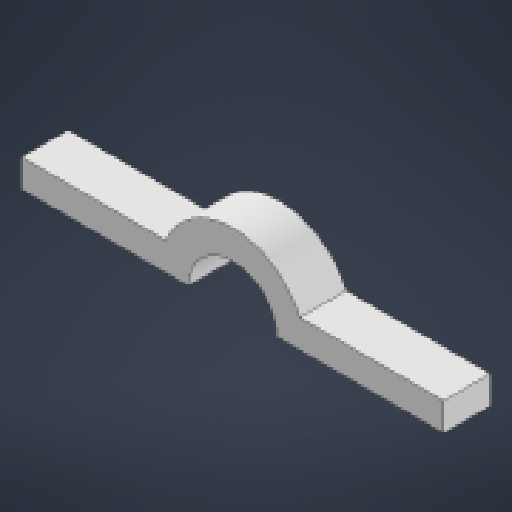
# Autodesk Inventor part: Idler-Clamp
Saved by Autodesk Inventor 2025 (Build 290162010, 162A)
## iProperties
Created: 2025-12-05
Part Number: Idler-Clamp
Material: Generic
Document SubType Name: Modeling
Designer: FizzyApple12
Density: 1 g/cm^3
Appearance: Default
Author: FizzyApple12
Autodesk Inventor part; units mm, degrees
ref_plane "YZ Plane" through (0, 0, 0) normal (1, 0, 0) x (0, 1, 0)
ref_plane "XZ Plane" through (0, 0, 0) normal (0, 1, 0) x (-1, 0, 0)
ref_plane "XY Plane" through (0, 0, 0) normal (0, 0, 1) x (1, 0, 0)
sketch "Sketch1" plane through (0, 0, 0) normal (0, 0, 1) x (1, 0, 0)
  circle A0 centre (0, 0) radius 6.15
  line L0 (-31.1793, -0.1) -> (31.1793, -0.1)
  line L1 (31.1793, -0.1) -> (31.1793, 0.1)
  line L2 (31.1793, 0.1) -> (-31.1793, 0.1)
  line L3 (-31.1793, 0.1) -> (-31.1793, -0.1)
  line L4 (-31.1793, -0.1) -> (31.1793, 0.1) construction
  line L5 (31.1793, -0.1) -> (-31.1793, 0.1) construction
  line L6 (-18, 4) -> (18, 4)
  line L7 (18, 4) -> (18, 0)
  line L8 (18, 0) -> (-18, 0)
  line L9 (-18, 0) -> (-18, 4)
  circle A1 centre (0, 0) radius 10.15
  line L10 (0, 0) -> (0, 10.15) construction
  line L11 (-14, 0) -> (14, 0) construction
  point P0 (0, 6.15)
  point P1 (18, 0.1)
  point P2 (9.3286, 4)
  point P3 (-9.3286, 4)
  point P4 (-18, 0.1)
  point P5 (-6.1492, 0.1)
  point P6 (6.1492, 0.1)
  dimension "d0" = 12.3
  dimension "d1" = 0.2
  dimension "d2" = 4
  dimension "d3" = 4
  dimension "d6" = 28
  dimension "d7" = 4
  constraints: 24 end point, 4 coincident, 4 midpoint, 4 parallel, 3 horizontal, 3 perpendicular, 1 point on line, 6 other
  measures "d1" distance of L1.end L0.end
  measures "d2" distance between parallel lines of L6 L8
  measures "d3" distance of L10.end point (0, 6.15)
  measures "d6" distance of L11.start L11.end
  measures "d7" distance from line of L7 L11.end
extrude "Extrusion1" add sketch "Sketch1" along normal blind 6.5 contours A0 L6 A1 L2 | A0 L6 A1 | A1 L6 L7 L2 | L2 A1 L6 A0 | L2 L9 L6 A1
sketch "Sketch2" plane through (9.3286, 4, 0) normal (0, 1, 0) x (1, 0, 0)
  line L0 (-18.6572, 0) -> (-18.6572, -6.5) construction
  line L1 (0, 0) -> (0, -6.5) construction
  line L2 (0, -3.25) -> (4.6714, -3.25) construction
  line L3 (-18.6572, -3.25) -> (-23.3286, -3.25) construction
  point P0 (-9.3286, 0)
  dimension "d8" = 28
  constraints: 4 end point, 2 coincident, 2 horizontal, 2 midpoint, 1 collinear
  measures "d8" distance of point (-23.329, -3.25) point (4.671, -3.25)
hole "Hole1" at (-14, 4, 3.25) at (14, 4, 3.25) direction (0, -1, 0) diameter 3.4 depth 8 clearance for "Flat Head Machine Screw" size "M3" standard "Ansi Metric M Profile"
fillet "Fillet1" radius 2 6 edges at (-18, 2.05, 0) (-18, 2.05, 6.5) (18, 2.05, 0) (18, 2.05, 6.5) (9.3286, 4, 3.25) (-9.3286, 4, 3.25)
chamfer "Chamfer1" distance 0.25 angle 45 33 edges at (0, 10.15, 6.5) (-9.559, 4.2715, 6.5) (-13.2826, 4, 6.5) (-17.4142, 4, 5.9142) (-18, 4, 3.25) (-17.4142, 4, 0.5858) (-13.2826, 4, 0) (-9.559, 4.2715, 0) (0, 10.15, 0) (9.559, 4.2715, 0) (13.2826, 4, 0) (17.4142, 4, 0.5858) (18, 4, 3.25) (17.4142, 4, 5.9142) (13.2826, 4, 6.5) (9.559, 4.2715, 6.5) (0, 6.15, 6.5) (-11.0746, 0.1, 6.5) (-17.4142, 0.1, 5.9142) (-18, 0.1, 3.25) (-17.4142, 0.1, 0.5858) (-11.0746, 0.1, 0) (11.0746, 0.1, 6.5) (17.4142, 0.1, 5.9142) (18, 0.1, 3.25) (17.4142, 0.1, 0.5858) (11.0746, 0.1, 0) (6.1492, 0.1, 3.25) (-6.1492, 0.1, 3.25) (14, 4, 1.55) (-14, 4, 1.55) (14, 0.1, 1.55) (-14, 0.1, 1.55)
body "Solid1"
